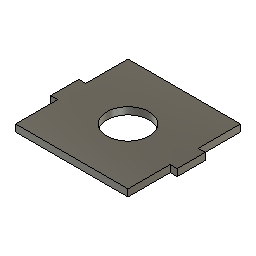
7thLesson v1 (Autodesk Fusion 360 design; units mm, degrees)
Autodesk Fusion 360 part; units mm, degrees
sketch "Sketch1" plane through (0, 0, 0) normal (0, 0, 1) x (1, 0, 0)
  line L0 (35, 60) -> (75, 60)
  line L1 (75, 60) -> (75, 45)
  line L2 (35, 60) -> (35, 45)
  line L3 (75, 45) -> (77.5, 45)
  line L4 (35, 45) -> (32.5, 45)
  line L5 (77.5, 45) -> (77.5, 35)
  line L6 (32.5, 45) -> (32.5, 35)
  line L7 (32.5, 35) -> (35, 35)
  line L8 (77.5, 35) -> (75, 35)
  line L9 (35, 35) -> (35, 20)
  line L10 (75, 35) -> (75, 20)
  line L11 (75, 20) -> (35, 20)
  circle A0 centre (55, 40) radius 7.5
  dimension "d1" = 40
  dimension "d2" = 15
  dimension "d3" = 15
  dimension "d4" = 2.5
  dimension "d5" = 2.5
  dimension "d6" = 10
  dimension "d7" = 10
  dimension "d8" = 2.5
  dimension "d9" = 2.5
  dimension "d10" = 15
  dimension "d11" = 15
  dimension "d12" = 15
  dimension "d13" = 20
  dimension "d14" = 22.5
  constraint horizontal L0
  constraint perpendicular L0 L1
  constraint perpendicular L0 L2
  constraint horizontal L3
  constraint horizontal L4
  constraint perpendicular L3 L5
  constraint perpendicular L4 L6
  constraint perpendicular L6 L7
  constraint perpendicular L5 L8
  constraint perpendicular L7 L9
  constraint perpendicular L8 L10
  measures "d1" distance of L0.start L0.end
  measures "d2" distance of L0.end L1.end
  measures "d3" distance of L0.start L2.end
  measures "d4" distance of L1.end L3.end
  measures "d5" distance of L2.end L4.end
  measures "d6" distance of L3.end L5.end
  measures "d7" distance of L4.end L6.end
  measures "d8" distance of L6.end L7.end
  measures "d9" distance of L5.end L8.end
  measures "d10" distance of L7.end L9.end
  measures "d11" distance of L8.end L10.end
  measures "d12" diameter of A0
  measures "d13" distance of L0 A0.centre
  measures "d14" distance of L5 A0.centre
extrude "Extrude1" add sketch "Sketch1" along normal blind 2.5
